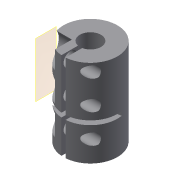
# Autodesk Inventor part: 00_Motorcoupling_5mm_M3_clamped
Saved by Autodesk Inventor 2022 (Build 260153000, 153)
## iProperties
Created: 2021-11-15
Part Number: 00_Motorcoupling_5mm_M3_clamped
Material: Generic
Document SubType Name: Modeling
Designer: diederichbenedict
Density: 1 g/cm^3
Appearance: Default
Author: diederichbenedict
Autodesk Inventor part; units mm, degrees
ref_plane "YZ Plane" through (0, 0, 0) normal (1, 0, 0) x (0, 1, 0)
ref_plane "XZ Plane" through (0, 0, 0) normal (0, 1, 0) x (-1, 0, 0)
ref_plane "XY Plane" through (0, 0, 0) normal (0, 0, 1) x (1, 0, 0)
sketch "Sketch1" plane through (0, 0, 0) normal (0, 1, 0) x (-1, 0, 0)
  circle A0 centre (0, 0) radius 1.55
  circle A1 centre (0, 0) radius 6.5
  dimension "d0" = 3.1
  dimension "d1" = 13
  constraints: 2 centre point, 2 coincident
  measures "d0" diameter of A0
  measures "d1" diameter of A1
extrude "Extrusion1" add sketch "Sketch1" along normal blind 8
sketch "Sketch2" plane through (0, 8, 0) normal (0, 1, 0) x (1, 0, 0)
  circle A0 centre (0, 0) radius 6.5 projected
  circle A1 centre (0, 0) radius 1.55 projected
  circle A2 centre (0, 0) radius 1.55 projected
  line L0 (-1.5265, 0.2692) -> (-6.4013, 1.1287)
  line L1 (1.5265, 0.2692) -> (6.4013, 1.1287)
  line L2 (-9.1, 0) -> (9.1, 0) projected
  line L3 (9.1, 0) -> (-9.1, 0) projected
  dimension "d6" = 10
  dimension "d7" = 10
  constraints: 4 end point, 4 point on circle, 2 line through centre
  measures "d6" angle of L2 L0
  measures "d7" angle of L1 L2
extrude "Extrusion2" add sketch "Sketch2" along normal blind 1 contours L1 A1 L0 A0
sketch "Sketch3" plane through (0, 9, 0) normal (0, 1, 0) x (1, 0, 0)
  arc A0 (6.4013, 1.1287) -> (-6.4013, 1.1287) centre (0, 0) ccw projected
  line L0 (-6.4013, 1.1287) -> (-1.5265, 0.2692) projected
  arc A1 (1.5265, 0.2692) -> (-1.5265, 0.2692) centre (0, 0) ccw projected
  line L1 (1.5265, 0.2692) -> (6.4013, 1.1287) projected
  circle A2 centre (0, 0) radius 1.55 projected
  circle A3 centre (0, 0) radius 2.55
  circle A4 centre (0, 0) radius 6.5
  point P0 (-6.4013, 1.1287)
  dimension "d10" = 5.1
  constraints: 2 centre point, 1 coincident, 1 concentric
  measures "d10" diameter of A3
extrude "Extrusion3" add sketch "Sketch3" along normal blind 12 contours L1 A3 L0 A0 | A4 L0 A3 L1 | A3 L0 A2 L1 | L1 A1 L0 A3
sketch "Sketch4" plane through (0, 21, 0) normal (0, 1, 0) x (1, 0, 0)
  circle A0 centre (0, 0) radius 6.5 projected
  circle A1 centre (0, 0) radius 1.55 projected
  line L0 (0.5, -0.9294) -> (-0.5, -0.9294)
  line L1 (-0.5, -0.9294) -> (-0.5, -14.8183)
  line L2 (-0.5, -14.8183) -> (0.5, -14.8183)
  line L3 (0.5, -14.8183) -> (0.5, -0.9294)
  line L4 (0.5, -0.9294) -> (-0.5, -14.8183) construction
  line L5 (-0.5, -0.9294) -> (0.5, -14.8183) construction
  point P0 (0, -7.8739)
  dimension "d13" = 1
  constraints: 12 end point, 2 midpoint, 2 parallel, 1 horizontal, 1 perpendicular
  measures "d13" distance between parallel lines of L3 L1
extrude "Extrusion4" cut sketch "Sketch4" against normal through all contours L1 A1 L3 A0 | A0 L3 L2 L1 | L1 L0 L3 A1 picked at (-0.0556, -3.1931) picked at (0.0565, -1.1332)
ref_plane "Work Plane1" through (-6.5, 21, 6.4807) normal (1, 0, 0) x (0, 0, -1)
sketch "Sketch5" plane through (-6.5, 21, 6.4807) normal (1, 0, 0) x (0, 0, -1)
  line L0 (0, -13) -> (0, -21) projected
  line L1 (0, -21) -> (0, -21) projected
  line L2 (0, -21) -> (0, -13) projected
  line L3 (7.6095, -13) -> (0, -13) projected
  line L4 (7.6095, -13) -> (7.6095, -12) projected
  line L5 (7.6095, -12) -> (0, -12) projected
  line L6 (0, -12) -> (0, 0) projected
  line L7 (0, 0) -> (0, 0) projected
  line L8 (0, 0) -> (0, -12) projected
  line L9 (0, -12) -> (7.6095, -12) projected
  line L10 (7.6095, -13) -> (7.6095, -12) projected
  line L11 (0, -13) -> (7.6095, -13) projected
  point P0 (6.4807, -21)
  point P1 (2.2189, -1.921)
hole "Hole1" at (-6.5, 19.079, 4.2619) direction (1, 0, 0) diameter 2.8 depth 12 tip angle 115 counterbore diameter 6 counterbore depth 4
pattern_linear "Rectangular Pattern1" count 3 spacing 7 along (0, -1, 0) of "Hole1"
sketch "Sketch6" plane through (0, 21, 0) normal (0, 1, 0) x (1, 0, 0)
  arc A0 (0.5, -1.4671) -> (-0.5, -1.4671) centre (0, 0) ccw projected
  circle A1 centre (0, 0) radius 2.55
  dimension "d27" = 5.1
  constraints: 1 centre point, 1 coincident
  measures "d27" diameter of A1
extrude "Extrusion5" cut sketch "Sketch6" against normal blind 12
sketch "Sketch7" plane through (-2.5, 12.079, 4.2619) normal (-1, 0, 0) x (0, 0, 1)
  circle A0 centre (0, -7) radius 1.4 projected
  line L0 (-0.6839, -4.079) -> (0.6839, -4.079) projected
  arc A1 (-0.6839, -4.079) -> (1.7381, -9.4452) centre (0, -7) ccw projected
  line L1 (1.7381, -4.5548) -> (1.7381, -9.4452) projected
  arc A2 (1.7381, -4.5548) -> (0.6839, -4.079) centre (0, -7) ccw projected
  line L2 (1.7381, 2.4452) -> (1.7381, -2.4452) projected
  arc A3 (1.7381, 2.4452) -> (1.7381, -2.4452) centre (0, 0) ccw projected
  circle A4 centre (0, 0) radius 1.4 projected
  circle A5 centre (0, 7) radius 1.4 projected
  line L3 (1.7381, 8.921) -> (1.7381, 4.5548) projected
  line L4 (-2.3043, 8.921) -> (1.7381, 8.921) projected
  arc A6 (-2.3043, 8.921) -> (1.7381, 4.5548) centre (0, 7) ccw projected
  circle A7 centre (0, 7) radius 1.4 projected
  circle A8 centre (0, -7) radius 1.6941
  circle A9 centre (0, 0) radius 1.4 projected
  circle A10 centre (0, 0) radius 1.7381
  circle A11 centre (0, 7) radius 1.7166
  point P0 (-4.2619, -12.079)
  point P1 (-1.2598, -0.6107)
  point P2 (-1.2598, 0.6107)
  constraints: 3 centre point, 3 coincident, 1 tangent
extrude "Extrusion6" cut sketch "Sketch7" against normal blind 3 contours A0 | A10 | A4 | A5 | A8 | A11
body "Solid1"
